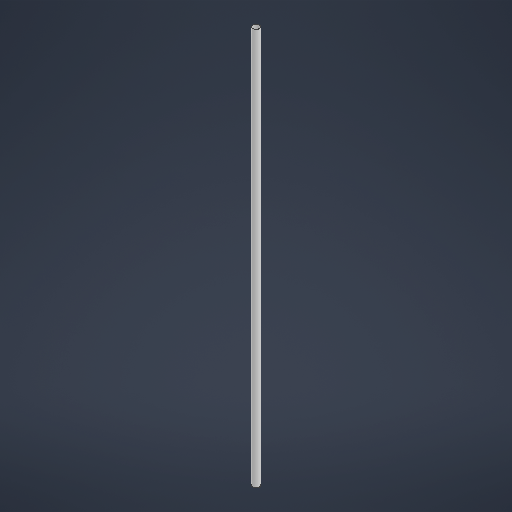
# Autodesk Inventor part: pole_v1
Saved by Autodesk Inventor 2026.2 (Build 302298000, 298)
## iProperties
Created: 2025-12-19
Part Number: pole_v1
Material: Generic
Document SubType Name: Modeling
Designer: colin
Density: 1 g/cm^3
Appearance: Default
Author: colin
Autodesk Inventor part; units mm, degrees
ref_plane "YZ Plane" through (0, 0, 0) normal (1, 0, 0) x (0, 1, 0)
ref_plane "XZ Plane" through (0, 0, 0) normal (0, 1, 0) x (-1, 0, 0)
ref_plane "XY Plane" through (0, 0, 0) normal (0, 0, 1) x (1, 0, 0)
sketch "Sketch3" plane through (0, 0, 0) normal (0, 1, 0) x (-1, 0, 0)
  circle A0 centre (0, 0) radius 12.775
  circle A1 centre (0, 0) radius 12.275
  dimension "d5" = 25.55
  dimension "d6" = 0.5
  constraints: 2 centre point, 1 coincident
  measures "d5" diameter of A0
  measures "d6" radial gap between concentric circles of A1 A0
extrude "Extrusion3" add sketch "Sketch3" along normal blind 1524
body "Solid2"
